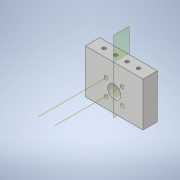
# Autodesk Inventor part: Y screw bracket
Saved by Autodesk Inventor 2020 (Build 240168000, 168)
## iProperties
Created: 2019-02-27
Part Number: Y screw bracket
Material: Generic
Document SubType Name: Modeling
Designer: LillaHunden
Density: 1 g/cm^3
Appearance: Default
Author: LillaHunden
Autodesk Inventor part; units mm, degrees
ref_plane "YZ Plane" through (0, 0, 0) normal (1, 0, 0) x (0, 1, 0)
ref_plane "XZ Plane" through (0, 0, 0) normal (0, 1, 0) x (-1, 0, 0)
ref_plane "XY Plane" through (0, 0, 0) normal (0, 0, 1) x (1, 0, 0)
sketch "Sketch1" plane through (0, 0, 0) normal (0, 0, 1) x (1, 0, 0)
  line L0 (-30.1791, 10) -> (-70.1791, 10)
  line L1 (-70.1791, 10) -> (-70.1791, 45)
  line L2 (-70.1791, 45) -> (-30.1791, 45)
  line L3 (-30.1791, 45) -> (-30.1791, 10)
  point P0 (0, 0)
  dimension "d0" = 40
  dimension "d1" = 35
  constraints: 8 end point, 2 parallel, 1 horizontal, 1 perpendicular
  measures "d0" distance of L1.end L2.end
  measures "d1" distance of L0.end L1.end
extrude "Extrusion1" add sketch "Sketch1" along normal blind 10
ref_plane "Work Plane1" through (-50.1791, 10, 0) normal (-1, 0, 0) x (0, 0, 1)
sketch "Sketch2" plane through (0, 0, 0) normal (0, 0, -1) x (-1, 0, 0)
  circle A0 centre (50.1791, 23) radius 4.5 projected
  point P0 (0, 0)
extrude "Extrusion2" cut sketch "Sketch2" against normal through all
sketch "Sketch3" plane through (0, 0, 0) normal (0, 0, -1) x (-1, 0, 0)
  circle A0 centre (50.1791, 23) radius 11 construction
  spline S0 degree 4 poles (51.7186, 14.1946) (51.6177, 14.2378) (51.4846, 14.315) (51.3291, 14.4434) (51.1731, 14.633) (51.0783, 14.7842) (51.0035, 14.9466) (50.9509, 15.1162) (50.9221, 15.2903) (50.9169, 15.4691) (50.9344, 15.6484) (50.9739, 15.8255) (51.0345, 15.998) (51.1442, 16.2221) (51.264, 16.3859) (51.375, 16.5007) (51.4557, 16.5626) knots 0 0 0 0 0 0.155358 0.217814 0.280385 0.342893 0.405256 0.467588 0.529988 0.592596 0.655528 0.718682 0.781929 0.845129 1 1 1 1 1 construction
  arc A1 (53.4951, 16.3178) -> (51.4555, 16.5624) centre (52.3382, 15.2969) ccw construction
  spline S1 degree 4 poles (53.4951, 16.3178) (53.5621, 16.2269) (53.6424, 16.09) (53.7201, 15.8998) (53.773, 15.6545) (53.7902, 15.4741) (53.7855, 15.294) (53.7588, 15.1165) (53.7101, 14.9462) (53.6385, 14.7843) (53.5451, 14.6315) (53.4329, 14.4918) (53.3037, 14.3673) (53.1072, 14.2209) (52.9284, 14.1357) (52.7792, 14.0918) (52.6795, 14.0793) knots 0 0 0 0 0 0.157528 0.220644 0.283729 0.346671 0.409336 0.471776 0.534146 0.596535 0.659071 0.721753 0.784393 0.846862 1 1 1 1 1 construction
  arc A2 (51.7186, 14.1946) -> (52.6506, 13.9518) centre (55.9524, 28.5379) ccw construction
  spline S2 degree 4 poles (57.2626, 24.0568) (57.1618, 24.1) (57.0288, 24.1775) (56.8733, 24.3059) (56.7176, 24.4958) (56.6229, 24.6472) (56.5483, 24.8098) (56.4959, 24.9796) (56.4672, 25.1538) (56.4621, 25.3326) (56.4796, 25.5121) (56.5191, 25.689) (56.5796, 25.8615) (56.689, 26.0852) (56.8086, 26.2487) (56.9193, 26.3632) (56.9997, 26.4248) knots 0 0 0 0 0 0.15539 0.217866 0.280459 0.342995 0.40539 0.467755 0.530187 0.592819 0.655765 0.718917 0.782144 0.845307 1 1 1 1 1 construction
  arc A3 (59.0391, 26.1801) -> (56.9995, 26.4247) centre (57.8822, 25.1591) ccw construction
  spline S3 degree 4 poles (59.0391, 26.1801) (59.1062, 26.0892) (59.1863, 25.9523) (59.2641, 25.7621) (59.317, 25.5168) (59.3341, 25.3364) (59.3295, 25.1562) (59.3029, 24.9788) (59.2541, 24.8084) (59.1825, 24.6466) (59.0891, 24.4937) (58.9769, 24.3541) (58.8477, 24.2295) (58.6513, 24.0832) (58.4723, 23.9979) (58.3232, 23.9541) (58.2235, 23.9415) knots 0 0 0 0 0 0.157519 0.220636 0.283723 0.346665 0.409333 0.471776 0.534144 0.596533 0.659072 0.721755 0.784397 0.846867 1 1 1 1 1 construction
  arc A4 (57.2626, 24.0568) -> (57.3357, 24.2574) centre (44.6412, 28.7733) ccw construction
  spline S4 degree 4 poles (47.4003, 29.6009) (47.2994, 29.644) (47.1664, 29.7212) (47.0108, 29.8495) (46.8548, 30.0392) (46.7601, 30.1905) (46.6852, 30.3529) (46.6327, 30.5226) (46.6038, 30.6967) (46.5987, 30.8756) (46.6162, 31.055) (46.6557, 31.2321) (46.7163, 31.4046) (46.826, 31.6286) (46.9458, 31.7923) (47.0568, 31.9071) (47.1374, 31.9688) knots 0 0 0 0 0 0.155355 0.217813 0.280388 0.342902 0.405274 0.467617 0.530028 0.592644 0.655582 0.718737 0.781979 0.845171 1 1 1 1 1 construction
  arc A5 (49.1769, 31.7241) -> (47.1373, 31.9687) centre (48.02, 30.7031) ccw construction
  spline S5 degree 4 poles (49.1769, 31.7241) (49.2439, 31.6332) (49.324, 31.4962) (49.4019, 31.306) (49.4548, 31.0607) (49.4719, 30.8803) (49.4673, 30.7002) (49.4406, 30.5228) (49.3918, 30.3524) (49.3203, 30.1906) (49.2269, 30.0378) (49.1147, 29.8981) (48.9854, 29.7735) (48.789, 29.6272) (48.6101, 29.542) (48.4609, 29.4981) (48.3612, 29.4855) knots 0 0 0 0 0 0.15753 0.22065 0.283735 0.346677 0.40934 0.471779 0.534146 0.596533 0.659069 0.721751 0.784392 0.846863 1 1 1 1 1 construction
  arc A6 (47.4003, 29.6009) -> (48.3129, 29.3386) centre (44.4058, 17.4621) ccw construction
  spline S6 degree 4 poles (41.8563, 19.7386) (41.7557, 19.7811) (41.6229, 19.8578) (41.4675, 19.9854) (41.3117, 20.1747) (41.2169, 20.3259) (41.142, 20.4885) (41.0893, 20.6584) (41.0602, 20.8328) (41.0549, 21.012) (41.0721, 21.1919) (41.1114, 21.3693) (41.1719, 21.5422) (41.2815, 21.7665) (41.4014, 21.9303) (41.5126, 22.045) (41.5934, 22.1066) knots 0 0 0 0 0 0.155069 0.21746 0.28 0.342515 0.404914 0.467305 0.529776 0.592454 0.655449 0.718651 0.781927 0.845142 1 1 1 1 1 construction
  arc A7 (43.6329, 21.8619) -> (41.5933, 22.1065) centre (42.476, 20.8409) ccw construction
  spline S7 degree 4 poles (43.6329, 21.8619) (43.6999, 21.7709) (43.7801, 21.634) (43.8578, 21.4438) (43.9108, 21.1985) (43.9279, 21.0181) (43.9233, 20.8379) (43.8966, 20.6605) (43.8478, 20.4902) (43.7763, 20.3283) (43.6828, 20.1755) (43.5707, 20.0359) (43.4414, 19.9113) (43.245, 19.765) (43.0661, 19.6798) (42.9169, 19.6359) (42.8172, 19.6233) knots 0 0 0 0 0 0.157535 0.220652 0.283739 0.34668 0.409345 0.471783 0.534148 0.596532 0.659068 0.721748 0.784389 0.84686 1 1 1 1 1 construction
  arc A8 (41.8563, 19.7386) -> (41.8675, 19.7997) centre (55.717, 17.2267) ccw construction
  circle A9 centre (50.1791, 23) radius 4.5 construction
  point P0 (0, 0)
  point P1 (51.5636, 14.2745)
  point P2 (51.4205, 14.3762)
  point P3 (51.2906, 14.4978)
  point P4 (51.1771, 14.6357)
  point P5 (51.0823, 14.7868)
  point P6 (51.0079, 14.9487)
  point P7 (50.9558, 15.1174)
  point P8 (50.9271, 15.2903)
  point P9 (50.9216, 15.4679)
  point P10 (50.9388, 15.6469)
  point P11 (50.9781, 15.8238)
  point P12 (51.0386, 15.9962)
  point P13 (51.119, 16.1604)
  point P14 (51.2178, 16.313)
  point P15 (51.3334, 16.4513)
  point P16 (53.5928, 16.1664)
  point P17 (53.6713, 16.0038)
  point P18 (53.7302, 15.8318)
  point P19 (53.7687, 15.6535)
  point P20 (53.7857, 15.4733)
  point P21 (53.7809, 15.2935)
  point P22 (53.754, 15.117)
  point P23 (53.7053, 14.9479)
  point P24 (53.6343, 14.7869)
  point P25 (53.5415, 14.6347)
  point P26 (53.4295, 14.4951)
  point P27 (53.3004, 14.3707)
  point P28 (53.1565, 14.2638)
  point P29 (53.0015, 14.1776)
  point P30 (52.8383, 14.1143)
  point P31 (57.1078, 24.1369)
  point P32 (56.9647, 24.2387)
  point P33 (56.8349, 24.3604)
  point P34 (56.7215, 24.4985)
  point P35 (56.627, 24.6498)
  point P36 (56.5527, 24.8119)
  point P37 (56.5007, 24.9807)
  point P38 (56.4722, 25.1538)
  point P39 (56.4668, 25.3315)
  point P40 (56.4841, 25.5105)
  point P41 (56.5233, 25.6874)
  point P42 (56.5837, 25.8597)
  point P43 (56.664, 26.0237)
  point P44 (56.7626, 26.1761)
  point P45 (56.8778, 26.314)
  point P46 (59.1367, 26.0287)
  point P47 (59.2153, 25.8661)
  point P48 (59.2742, 25.6941)
  point P49 (59.3127, 25.5159)
  point P50 (59.3296, 25.3356)
  point P51 (59.3249, 25.1557)
  point P52 (59.298, 24.9793)
  point P53 (59.2493, 24.8101)
  point P54 (59.1783, 24.6491)
  point P55 (59.0855, 24.497)
  point P56 (58.9735, 24.3574)
  point P57 (58.8443, 24.2329)
  point P58 (58.7005, 24.126)
  point P59 (58.5455, 24.0398)
  point P60 (58.3823, 23.9765)
  point P61 (47.2454, 29.6807)
  point P62 (47.1022, 29.7824)
  point P63 (46.9723, 29.9039)
  point P64 (46.8588, 30.0419)
  point P65 (46.7641, 30.1931)
  point P66 (46.6896, 30.3551)
  point P67 (46.6376, 30.5237)
  point P68 (46.6089, 30.6968)
  point P69 (46.6034, 30.8745)
  point P70 (46.6206, 31.0535)
  point P71 (46.6599, 31.2304)
  point P72 (46.7204, 31.4028)
  point P73 (46.8008, 31.5669)
  point P74 (46.8996, 31.7195)
  point P75 (47.0152, 31.8577)
  point P76 (49.2745, 31.5727)
  point P77 (49.353, 31.41)
  point P78 (49.412, 31.238)
  point P79 (49.4504, 31.0598)
  point P80 (49.4674, 30.8795)
  point P81 (49.4626, 30.6997)
  point P82 (49.4358, 30.5233)
  point P83 (49.3871, 30.3541)
  point P84 (49.3161, 30.1932)
  point P85 (49.2233, 30.041)
  point P86 (49.1113, 29.9015)
  point P87 (48.9821, 29.7769)
  point P88 (48.8383, 29.67)
  point P89 (48.6833, 29.5839)
  point P90 (48.5201, 29.5205)
  point P91 (41.7018, 19.8176)
  point P92 (41.5589, 19.9186)
  point P93 (41.4292, 20.0396)
  point P94 (41.3157, 20.1773)
  point P95 (41.221, 20.3284)
  point P96 (41.1464, 20.4905)
  point P97 (41.0942, 20.6594)
  point P98 (41.0653, 20.8328)
  point P99 (41.0595, 21.0109)
  point P100 (41.0766, 21.1903)
  point P101 (41.1156, 21.3676)
  point P102 (41.176, 21.5404)
  point P103 (41.2564, 21.7048)
  point P104 (41.3552, 21.8575)
  point P105 (41.4709, 21.9956)
  point P106 (43.7305, 21.7104)
  point P107 (43.809, 21.5477)
  point P108 (43.868, 21.3758)
  point P109 (43.9064, 21.1975)
  point P110 (43.9234, 21.0173)
  point P111 (43.9186, 20.8374)
  point P112 (43.8918, 20.661)
  point P113 (43.843, 20.4919)
  point P114 (43.7721, 20.3309)
  point P115 (43.6793, 20.1788)
  point P116 (43.5673, 20.0392)
  point P117 (43.4381, 19.9147)
  point P118 (43.2943, 19.8078)
  point P119 (43.1393, 19.7216)
  point P120 (42.9761, 19.6583)
  constraints: 16 point on circle, 10 centre point, 4 coincident, 136 other
hole "Hole1" at (-44.6412, 28.7733, 0) at (-44.4058, 17.4621, 0) at (-55.717, 17.2267, 0) at (-55.9524, 28.5379, 0) direction (0, 0, 1) diameter 2.459 end through all thread size "M3x0.5" class "6H" standard "ISO Metric profile"
sketch "Sketch4" plane through (-70.1791, 45, 0) normal (0, 1, 0) x (1, 0, 0)
  line L0 (0, 0) -> (0, -10) construction
  line L1 (0, -5) -> (40, -5) construction
  line L2 (40, 0) -> (40, -10) construction
  point P0 (70.1791, 0)
  point P1 (8, -5)
  point P2 (16, -5)
  point P3 (24, -5)
  point P4 (32, -5)
  dimension "d13" = 8
  dimension "d14" = 8
  dimension "d15" = 8
  dimension "d33" = 8
  dimension "d34" = 8
  constraints: 4 point on line, 2 end point, 2 midpoint
  measures "d13" distance from line of L0 point (8, -5)
  measures "d14" distance of point (16, -5) point (8, -5)
  measures "d15" distance of point (24, -5) point (16, -5)
  measures "d33" distance of point (24, -5) point (32, -5)
  measures "d34" distance of L1.end point (32, -5)
move faces "Move1" translate (0, -4.35, 0) faces at (-56.8458, 45, 3.3333)
hole "Hole3" at (-62.1791, 45, 5) at (-54.1791, 45, 5) at (-46.1791, 45, 5) at (-38.1791, 45, 5) direction (0, -1, 0) diameter 2.459 depth 8.8 tip angle 118 thread size "M3x0.5" class "6H" standard "ISO Metric profile"
equation "\"d14\" = d13"
equation "\"d15\" = d14"
equation "\"d33\" = d15"
body "Solid1"
